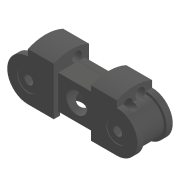
# Autodesk Inventor part: Middle
Saved by Autodesk Inventor 2020 (Build 240168000, 168)
## iProperties
Created: 2021-03-24
Part Number: Middle
Material: Generic
Document SubType Name: Modeling
Designer: deox
Density: 1 g/cm^3
Appearance: Generic
Author: deox
Autodesk Inventor part; units mm, degrees
sketch "Sketch1" plane through (0, 0, 0) normal (0, 0, 1) x (1, 0, 0)
  line L0 (-4.5, -4.075) -> (4.5, -4.075)
  line L1 (4.5, -4.075) -> (4.5, 4.075)
  line L2 (4.5, 4.075) -> (-4.5, 4.075)
  line L3 (-4.5, 4.075) -> (-4.5, -4.075)
  line L4 (-4.5, -4.075) -> (4.5, 4.075) construction
  line L5 (4.5, -4.075) -> (-4.5, 4.075) construction
  point P0 (0, 0)
  dimension "d0" = 9
  dimension "d1" = 8.15
  constraints: 12 end point, 2 midpoint, 2 parallel, 1 horizontal, 1 perpendicular
  measures "d0" distance of L2.end L1.end
  measures "d1" distance of L1.end L0.end
extrude "Extrusion1" add sketch "Sketch1" along normal blind 6.4
sketch "Sketch2" plane through (4.5, -4.075, 0) normal (1, 0, 0) x (0, 0, -1)
  line L0 (0, 8.15) -> (-6.4, 8.15) projected
  line L1 (-3.2, 8.15) -> (-3.2, 11.4)
  line L2 (-3.2, 8.15) -> (-7.45, 8.15)
  line L3 (-7.45, 8.15) -> (-7.45, -1.1)
  line L4 (0, 0) -> (-6.4, 0) projected
  line L5 (-5.9325, -1.1) -> (-5.9325, 0)
  line L6 (-7.45, -1.1) -> (-5.9325, -1.1)
  line L7 (-7.45, 8.15) -> (-7.45, 13.2689)
  line L8 (1.05, 8.15) -> (1.05, -1.1)
  line L9 (-0.4675, -1.1) -> (-0.4675, 0)
  line L10 (1.05, -1.1) -> (-0.4675, -1.1)
  line L11 (1.05, 8.15) -> (1.05, 13.2689)
  arc A0 (1.05, 10.4813) -> (-7.45, 10.4813) centre (-3.2, 1.1101) ccw
  line L12 (-7.45, 10.4813) -> (1.05, 10.4813) construction
  line L13 (-7.45, 10.4813) -> (1.05, 10.4813) construction
  point P0 (0, 4.075)
  point P1 (-0.4675, 0)
  dimension "d4" = 3.25
  dimension "d5" = 4.25
  dimension "d6" = 9.25
  dimension "d8" = 0
  constraints: 24 end point, 5 symmetric about line, 3 horizontal, 3 point on circle, 3 point on line, 3 vertical, 1 centre point, 1 collinear, 1 midpoint
  measures "d4" distance of L1.start L1.end
  measures "d5" distance of L1.start L2.end
  measures "d6" distance of L2.end L3.end
  measures "d8" distance between parallel lines of L12 L13
extrude "Extrusion2" add sketch "Sketch2" along normal blind 6.25
mirror "Mirror1" about plane through (0, 0, 0) normal (1, 0, 0) of "Extrusion2"
sketch "Sketch3" plane through (4.5, -5.175, 7.45) normal (0, 0, 1) x (1, 0, 0)
  line L0 (6.25, 0) -> (6.25, 11.5813) projected
  circle A0 centre (6.25, 5) radius 5
  line L1 (-4.5, 5.175) -> (-4.5, 2.6281)
  circle A1 centre (-15.25, 5) radius 5
  dimension "d11" = 10
  constraints: 2 end point, 1 centre point, 1 point on line, 1 symmetric about line, 1 vertical, 1 vertical alignment, 3 other
extrude "Extrusion3" add sketch "Sketch3" against normal up to surface (8.5 mm away)
sketch "Sketch4" plane through (0, 0, 0) normal (1, 0, 0) x (0, 1, 0)
  line L0 (-5.175, 5.9325) -> (-4.075, 5.9325) projected
  line L1 (-4.075, 5.9325) -> (-4.075, 0.4675) projected
  line L2 (-4.075, 0.4675) -> (-5.175, 0.4675) projected
  line L3 (-5.175, 7.45) -> (-5.175, 5.9325) projected
  line L4 (-5.175, 0.4675) -> (-5.175, -1.05) projected
  line L5 (-5.175, 5.9325) -> (-5.175, 0.4675)
  line L6 (-5.175, 0.4675) -> (-4.525, 0.4675)
  line L7 (-4.525, 0.4675) -> (-4.525, 5.9325)
  line L8 (-5.175, 5.9325) -> (-4.075, 5.9325) projected
  line L9 (-4.525, 5.9325) -> (-5.175, 5.9325)
  point P0 (0, 0)
  dimension "d25" = 0.65
  constraints: 8 end point, 2 perpendicular, 2 point on line, 1 collinear
  measures "d25" distance of L2.end L6.end
extrude "Extrusion4" cut sketch "Sketch4" against normal through all both and the other way through all contours L0 L7 L2 L5
sketch "Sketch5" plane through (4.5, -5.175, 7.45) normal (0, 0, 1) x (1, 0, 0)
  arc A0 (6.25, 0) -> (6.25, 10) centre (6.25, 5) ccw projected
  circle A1 centre (6.25, 5) radius 1.06
  line L0 (-4.5, 5.175) -> (-4.5, 8.0603)
  circle A2 centre (-15.25, 5) radius 1.06
  dimension "d16" = 2.12
  constraints: 2 centre point, 2 coincident, 2 end point, 2 symmetric about line, 1 vertical, 1 other
  measures "d16" diameter of A1
extrude "Extrusion5" cut sketch "Sketch5" against normal through all
ref_plane "Work Plane1" through (4.5, -5.175, 3.2) normal (0, 0, 1) x (1, 0, 0)
sketch "Sketch6" plane through (4.5, -5.175, 3.2) normal (0, 0, 1) x (1, 0, 0)
  circle A0 centre (6.25, 5) radius 1.06 projected
  arc A1 (3.1211, 1.1) -> (6.25, 10) centre (6.25, 5) ccw
  arc A2 (4.3232, 1.1) -> (6.25, 9.35) centre (6.25, 5) ccw
  line L0 (-4.5, 5.175) -> (-4.5, 10.9933)
  line L1 (0, 1.1) -> (3.1211, 1.1) projected
  line L2 (3.1211, 1.1) -> (4.3232, 1.1)
  arc A3 (6.25, 0) -> (6.25, 10) centre (6.25, 5) ccw projected
  line L3 (6.25, 10) -> (6.25, 9.35)
  line L4 (6.25, 10) -> (6.25, 11.5813) projected
  circle A4 centre (-15.25, 5) radius 1.06
  arc A5 (-15.25, 10) -> (-12.1211, 1.1) centre (-15.25, 5) ccw
  arc A6 (-15.25, 9.35) -> (-13.3232, 1.1) centre (-15.25, 5) ccw
  line L5 (-12.1211, 1.1) -> (-13.3232, 1.1)
  arc A7 (-15.25, 10) -> (-15.25, 0) centre (-15.25, 5) ccw
  line L6 (-15.25, 10) -> (-15.25, 9.35)
  dimension "d19" = 8.7
  constraints: 11 end point, 10 point on circle, 10 symmetric about line, 6 centre point, 4 coincident, 2 point on line, 1 collinear, 1 vertical, 4 other
  measures "d19" diameter of A2
extrude "Extrusion6" cut sketch "Sketch6" against normal mid plane 5.5 contours L2 A2 L3 A1 | L6 A6 L5 A5
sketch "Sketch7" plane through (0, 0, 6.4) normal (0, 0, 1) x (1, 0, 0)
  circle A0 centre (0, 0) radius 2.5
  dimension "d22" = 5
  constraints: 1 centre point, 1 coincident
  measures "d22" diameter of A0
extrude "Extrusion7" cut sketch "Sketch7" against normal through all
ref_plane "Work Plane2" through (-4.5, -5.175, 7.45) normal (-0.6428, -0.766, 0) x (0, 0, -1)
sketch "Sketch8" plane through (-4.5, -5.175, 7.45) normal (-0.6428, -0.766, 0) x (0, 0, -1)
  line L0 (7.45, 2.6208) -> (7.45, -2.3792) projected
  line L1 (1.05, -2.3792) -> (1.05, 2.6208) projected
  line L2 (1.05, 0.1208) -> (7.45, 0.1208)
  circle A0 centre (4.25, 0.1208) radius 1.5
  dimension "d27" = 3
  constraints: 2 end point, 2 midpoint, 1 centre point, 1 perpendicular
  measures "d27" diameter of A0
extrude "Extrusion8" cut sketch "Sketch8" against normal blind 5.5
ref_plane "Work Plane3" through (10.75, 4.175, 3.2) normal (0.9063, 0.4226, 0) x (0, 0, 1)
sketch "Sketch9" plane through (10.75, 4.175, 3.2) normal (0.9063, 0.4226, 0) x (0, 0, 1)
  line L0 (-3.2, -3.2593) -> (-3.2, 1.7407) projected
  line L1 (3.2, 1.7407) -> (3.2, -3.2593) projected
  circle A0 centre (1.5845, -0.0043) radius 1.15
  point P0 (-3.2, -0.7593)
  point P1 (0, 1.4454)
  dimension "d31" = 2.3
  constraints: 1 centre point, 1 other
  measures "d31" diameter of A0
extrude "Extrusion9" cut sketch "Sketch9" along normal blind 5.5 and the other way blind 11.25
sketch "Sketch10" plane through (-10.75, -2.9649, 3.2) normal (-1, 0, 0) x (0, 0, 1)
  circle A0 centre (-1.3656, 8.1157) radius 1.15
  point P0 (-3.2, 2.9649)
  dimension "d36" = 2.3
  constraints: 1 centre point
  measures "d36" diameter of A0
extrude "Extrusion10" cut sketch "Sketch10" against normal through all
sketch "Sketch11" plane through (-4.5, -5.175, 7.45) normal (0, 0, 1) x (1, 0, 0)
  circle A0 centre (-6.25, 5) radius 1.06 projected
  circle A1 centre (-6.25, 5) radius 2.575
  line L0 (4.5, 5.175) -> (4.5, 11.4443)
  circle A2 centre (15.25, 5) radius 2.575
  dimension "d39" = 5.15
  constraints: 2 centre point, 2 end point, 1 coincident, 1 symmetric about line, 1 vertical, 1 other
  measures "d39" diameter of A1
extrude "Extrusion11" cut sketch "Sketch11" against normal blind 0.2
mirror "Mirror2" about plane through (4.5, -5.175, 3.2) normal (0, 0, 1) of "Extrusion11"
body "Solid1"
